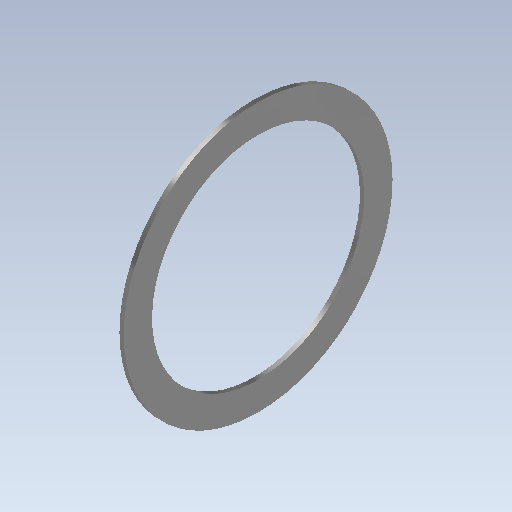
# Autodesk Inventor part: LF-1480ZZ_shield
Saved by Autodesk Inventor 2021 (Build 250183000, 183)
## iProperties
Created: 2019-07-28
Part Number: LF-1480ZZ_shield
Material: 鋼、炭素鋼
Catalog Web Link: www.cadenas.de
Description: Radial Flanged Ball Bearings (RF-Series/LF series) Metric ST shield-Radial Flanged Ball Bearings (RF-Series/LF series) Metric Shielded Type
Vendor: NMB
Document SubType Name: Modeling
Designer: psadmin
Manufacturer: NMB
Mass: 0.0733587 g
Surface Area: 1.07556 cm^2
Volume: 0.00934506 cm^3
Density: 7.85 g/cm^3
Appearance: 半つや出し
Category: PARTsolutions
Company: NMB
PSOL_IDENT_0: {$CADENAS_DATA\23d-libs\nmb\pbbp\radial_flanged_ball_bearings\rfbb_rflfs_m\rflf_shielded_shield.prj}
PSOL_IDENT_1: ,235 {VTYP=3D},{NB=LF-1480ZZ_shield},{LINA=LF-1480ZZ_shield},{NN=Radial Flanged Ball Bearings (RF-Se
PSOL_IDENT_2: ries/LF series) Metric ST shield},{DATE=11.11.2013 05:13:45},{GEOMDATE=24.10.2013 09:56:00},{VERSION=
PSOL_IDENT_3: },{LINEID=1270},{WBVAR=},{WBNUMERIC=}  {NB=LF-1480ZZ_shield},{LINA=LF-1480ZZ_shield},{KT=DUMMY},{IDN
PSOL_IDENT_4: R=},{PN=LF-1480ZZ},{SHLD=shielded},{FLANG=flanged},{SD=8.000},{D=14.000},{B=4.000},{SR=0.15},{BCZ=10
PSOL_IDENT_5: },{DW=1.5875},{LI=9.90},{LO=12.55},{D1=15.600},{C1=0.80},{D2=0.0},{C2=0.00},{COR=386},{CR=1036},{PCD=
PSOL_IDENT_6: 11.000},{U=12.588},{W=9.413},{Y=0.794},{Z=0.794},{AA=12.429},{AC=0.80},{AD=0.000},{AF=0.00},{AQ=0.20
PSOL_IDENT_7: },{AH=12.75},{AI=10.10},{AJ=0.40}
NN: Radial Flanged Ball Bearings (RF-Series/LF series) Metric ST shield
NT: Radial Flanged Ball Bearings (RF-Series/LF series) Metric Shielded Type
NB: LF-1480ZZ_shield
NBSYN: $PN._shield
LINA: LF-1480ZZ_shield
PN: LF-1480ZZ
SHLD: shielded
FLANG: flanged
SD: 8
D: 14
B: 4
SR: 0.15
BCZ: 10
DW: 1.5875
LI: 9.9
LO: 12.55
D1: 0
C1: 0.8
D2: 0
C2: 0
COR: 386
CR: 1036
PCD: 11
U: 12.588
W: 9.413
Y: 0.794
Z: 0.794
AA: 12.429
AC: 0.8
AD: 0
AF: 0
AQ: 0.2
AH: 12.75
AI: 10.1
AJ: 0.4
SUPPLIER: NMB
ARTICLENO: LF-1480ZZ_shield
BOMINFO: LF-1480ZZ_shield
CREATOR: CADENAS GmbH
Title: LF-1480ZZ_shield
Author: Cadenas PARTsolutions
Comments: Radial Flanged Ball Bearings (RF-Series/LF series) Metric Shielded Type
Autodesk Inventor part; units mm, degrees
sketch "Sketch_1" plane through (0, 0, 0) normal (0, 0, 1) x (1, 0, 0)
  line L0 (0.2, 0) -> (0, 0)
  line L1 (0, 6.275) -> (0, 4.95)
  line L2 (0, 4.95) -> (0.2, 4.95)
  line L3 (0.2, 4.95) -> (0.2, 6.275)
  line L4 (0.2, 6.275) -> (0, 6.275)
  constraints: 10 end point
revolve "Revolution1" add sketch "Sketch_1" angle 360 about axis through (0.2, 0, 0) along (1, 0, 0)
ref_plane "1_XY" through (0, 0, 0) normal (1, 0, 0) x (0, 0, -1)
ref_plane "1_YZ" through (0, 0, 0) normal (0, 0, -1) x (0, 1, 0)
ref_plane "1_ZX" through (0, 0, 0) normal (0, 1, 0) x (1, 0, 0)
body "Solid1"
